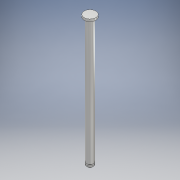
# Autodesk Inventor part: naprava
Saved by Autodesk Inventor 2018 (Build 220112000, 112)
## iProperties
Created: 2023-12-05
Part Number: naprava
Material: Všeobecné
Document SubType Name: Modeling
Designer: 42073
Density: 1 g/cm^3
Appearance: Hliník – leštěný
Author: 42073
Autodesk Inventor part; units mm, degrees
ref_plane "YZ Plane" through (0, 0, 0) normal (1, 0, 0) x (0, 1, 0)
ref_plane "XZ Plane" through (0, 0, 0) normal (0, 1, 0) x (-1, 0, 0)
ref_plane "XY Plane" through (0, 0, 0) normal (0, 0, 1) x (1, 0, 0)
sketch "Náčrt1" plane through (0, 0, 0) normal (0, 0, 1) x (1, 0, 0)
  circle A0 centre (0, 0) radius 1.5
  dimension "d0" = 3
  constraints: 1 centre point, 1 coincident
  measures "d0" diameter of A0
extrude "Vysunutí1" add sketch "Náčrt1" along normal blind 55.5
sketch "Náčrt2" plane through (0, 0, 55.5) normal (0, 0, 1) x (1, 0, 0)
  circle A0 centre (0, 0) radius 2.5
  dimension "d3" = 5
  constraints: 1 centre point, 1 coincident
  measures "d3" diameter of A0
extrude "Vysunutí2" add sketch "Náčrt2" along normal blind 1
sketch "Náčrt3" plane through (0, 0, 0) normal (0, 1, 0) x (-1, 0, 0)
  line L0 (-1.5, 0) -> (1.5, 0) projected
  line L1 (-1.5, 1) -> (-1, 1)
  line L2 (-1, 1) -> (-1, 1.5)
  line L3 (-1, 1.5) -> (-1.5, 1.5)
  line L4 (-1.5, 1.5) -> (-1.5, 1)
  point P0 (0, 0)
  dimension "d8" = 0.5
  dimension "d9" = 0.5
  dimension "d10" = 0.5
  constraints: 8 end point, 1 horizontal, 1 perpendicular
  measures "d8" distance of L1.start L1.end
  measures "d9" distance of L1.end L2.end
  measures "d10" distance of L2.end L3.end
sketch3d "3D náčrt1"
  arc A0 (1.5, 0, 0) -> (0, -1.5, 0) centre (0, 0, 0) ccw
  arc A1 (0, -1.5, 0) -> (-1.5, 0, 0) centre (0, 0, 0) ccw
  arc A2 (-1.5, 0, 0) -> (0, 1.5, 0) centre (0, 0, 0) ccw
  arc A3 (0, 1.5, 0) -> (1.5, 0, 0) centre (0, 0, 0) ccw
sweep "Tažení1" cut profiles "Náčrt3" path "3D náčrt1"
chamfer "Zkosení1" distance 0.5 angle 45 1 edges at (-1.5, 0, 0)
